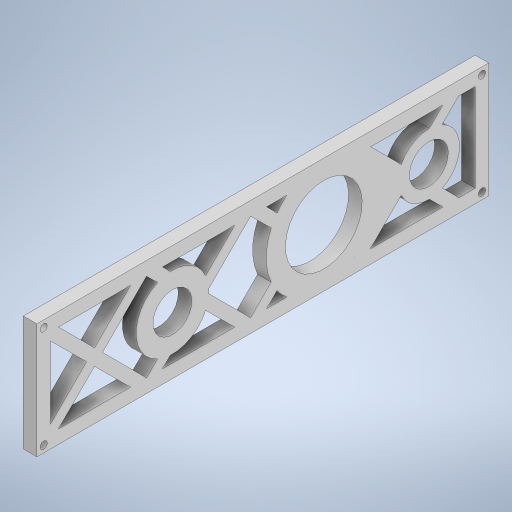
# Autodesk Inventor part: Side_Bracket
Saved by Autodesk Inventor 2023 (Build 270158030, 158C)
## iProperties
Created: 2022-06-17
Part Number: Side_Bracket
Material: Generic
Document SubType Name: Modeling
Designer: Mlees
Density: 1 g/cm^3
Appearance: Default
Author: Mlees
Autodesk Inventor part; units mm, degrees
ref_plane "YZ Plane" through (0, 0, 0) normal (1, 0, 0) x (0, 1, 0)
ref_plane "XZ Plane" through (0, 0, 0) normal (0, 1, 0) x (-1, 0, 0)
ref_plane "XY Plane" through (0, 0, 0) normal (0, 0, 1) x (1, 0, 0)
sketch "Sketch1" plane through (0, 0, 0) normal (1, 0, 0) x (0, 1, 0)
  line L0 (0, 0) -> (51, 0)
  line L1 (51, 0) -> (51, -200)
  line L2 (51, -200) -> (0, -200)
  line L3 (0, -200) -> (0, 0)
  circle A0 centre (25.5, -60) radius 8.625
  circle A1 centre (25.5, -173.5) radius 8.625
  line L4 (41.4645, -6) -> (9.5355, -6)
  line L5 (6, -194) -> (45, -194)
  line L6 (41.4645, -6) -> (25.5, -21.9645)
  line L7 (21.9645, -25.5) -> (6, -41.4645)
  line L8 (45, -41.4645) -> (29.0355, -25.5)
  line L9 (25.5, -21.9645) -> (9.5355, -6)
  line L10 (6, -9.5355) -> (21.9645, -25.5)
  line L11 (25.5, -29.0355) -> (45, -48.5355)
  line L12 (45, -9.5355) -> (29.0355, -25.5)
  line L13 (25.5, -29.0355) -> (7.7678, -46.7678)
  line L14 (45, -41.4645) -> (45, -9.5355)
  line L15 (7.7678, -46.7678) -> (6, -48.5355)
  line L16 (6, -9.5355) -> (6, -41.4645)
  line L17 (45, -73.625) -> (45, -55.6066)
  line L18 (6, -55.6066) -> (6, -73.625)
  line L19 (6, -73.625) -> (6, -87.5355)
  line L20 (45, -73.625) -> (45, -87.5355)
  line L21 (6, -48.5355) -> (10.8115, -53.347)
  line L22 (45, -48.5355) -> (40.1885, -53.347)
  line L23 (45, -55.6066) -> (43.7241, -56.8825)
  line L24 (43.7241, -56.8825) -> (41.5947, -59.0119)
  line L25 (6, -55.6066) -> (7.2759, -56.8825)
  line L26 (7.2759, -56.8825) -> (9.4053, -59.0119)
  arc A2 (40.1885, -53.347) -> (10.8115, -53.347) centre (25.5, -60) ccw
  line L27 (32.153, -74.6885) -> (45, -87.5355)
  arc A3 (32.153, -74.6885) -> (41.5947, -59.0119) centre (25.5, -60) ccw
  line L28 (18.847, -74.6885) -> (6, -87.5355)
  arc A4 (9.4053, -59.0119) -> (18.847, -74.6885) centre (25.5, -60) ccw
  arc A5 (24.5119, -76.0947) -> (26.4881, -76.0947) centre (25.5, -60) ccw
  line L29 (9.5355, -183.2132) -> (6, -186.7487)
  line L30 (41.4645, -183.1066) -> (45, -186.6421)
  line L31 (11.8783, -173.7994) -> (6, -179.6777)
  line L32 (39.1236, -173.6947) -> (45, -179.5711)
  line L33 (6, -147.6421) -> (19.5842, -161.2263)
  line L34 (37.7737, -179.4158) -> (41.4645, -183.1066)
  line L35 (45, -147.7487) -> (31.4876, -161.2612)
  line L36 (13.2612, -179.4876) -> (9.5355, -183.2132)
  arc A6 (19.5842, -161.2263) -> (11.8783, -173.7994) centre (25.5, -173.5) ccw
  arc A7 (13.2612, -179.4876) -> (37.7737, -179.4158) centre (25.5, -173.5) ccw
  arc A8 (39.1236, -173.6947) -> (31.4876, -161.2612) centre (25.5, -173.5) ccw
  line L37 (45, -194) -> (45, -186.6421)
  line L38 (45, -179.5711) -> (45, -147.7487)
  line L39 (6, -147.6421) -> (6, -179.6777)
  line L40 (6, -186.7487) -> (6, -194)
  circle A9 centre (25.5, -127) radius 17
  line L41 (6, -94.6066) -> (24.5119, -76.0947)
  line L42 (26.4881, -76.0947) -> (45, -94.6066)
  line L43 (6, -101.6777) -> (6, -110.5683)
  arc A10 (10.6165, -106.2942) -> (6, -110.5683) centre (25.5, -127) ccw
  line L44 (6, -94.6066) -> (15.1073, -103.7139)
  line L45 (6, -101.6777) -> (10.6165, -106.2942)
  line L46 (45, -94.6066) -> (35.8927, -103.7139)
  line L47 (45, -101.6777) -> (40.3835, -106.2942)
  line L48 (10.9259, -135.7518) -> (6, -140.6777)
  line L49 (2.5178, -137.0888) -> (2.2139, -137.3927)
  line L50 (6, -140.5711) -> (6.0533, -140.6244)
  line L51 (6, -143.4317) -> (6, -140.5711)
  arc A11 (35.8927, -103.7139) -> (15.1073, -103.7139) centre (25.5, -127) ccw
  line L52 (45, -101.6777) -> (45, -110.5683)
  arc A12 (6, -143.4317) -> (45, -143.4317) centre (25.5, -127) ccw
  arc A13 (45, -110.5683) -> (40.3835, -106.2942) centre (25.5, -127) ccw
  line L53 (40.0741, -135.7518) -> (45, -140.6777)
  line L54 (45, -143.4317) -> (45, -140.6777)
  point P0 (25.5, -200)
  dimension "d0" = 51
  dimension "d1" = 200
  dimension "d46" = 34
  constraints: 110 end point, 34 parallel, 24 point on circle, 14 centre point, 8 perpendicular, 5 vertical, 2 point on line, 1 coincident, 1 horizontal, 1 midpoint, 1 tangent
  measures "d0" distance of L1.end L2.end
  measures "d1" distance of L0.end L1.end
  measures "d46" diameter of A9
extrude "Extrusion1" add sketch "Sketch1" along normal blind 6 contours L0 L1 L2 L3 | A9 L53 L54 A12 L51 L48
sketch "Sketch4" plane through (6, 0, 0) normal (1, 0, 0) x (0, 0, -1)
  line L0 (200, 51) -> (0, 51) projected
  line L1 (0, 0) -> (200, 0) projected
  line L2 (0, 51) -> (0, 0) projected
  line L3 (200, 0) -> (200, 51) projected
  point P0 (3, 48)
  point P1 (197, 48)
  point P2 (3, 3)
  point P3 (197, 3)
hole "Hole1" at (6, 48, -3) at (6, 3, -3) at (6, 3, -197) at (6, 48, -197) direction (-1, 0, 0) diameter 3.25 end through all
body "Solid1"
